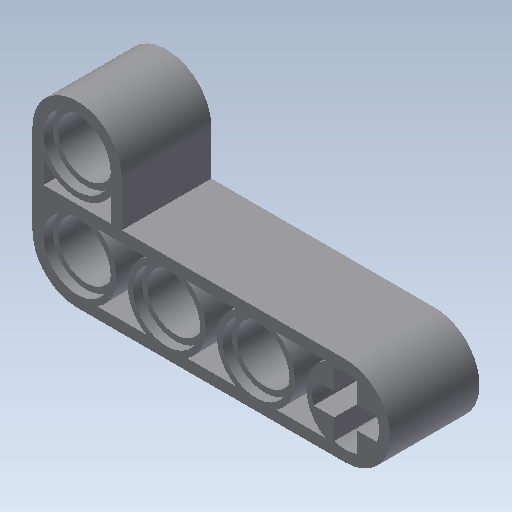
# Autodesk Inventor part: 5MRA Beam
Saved by Autodesk Inventor 2020 (Build 240168000, 168)
## iProperties
Created: 2014-02-14
Part Number: 5MRA Beam
Document SubType Name: Modeling
Designer: Jacob
Density: 1 g/cm^3
Material: Generic
Appearance: Default
Author: Jacob
Autodesk Inventor part; units mm, degrees
ref_plane "YZ Plane" through (0, 0, 0) normal (1, 0, 0) x (0, 1, 0)
ref_plane "XZ Plane" through (0, 0, 0) normal (0, 1, 0) x (-1, 0, 0)
ref_plane "XY Plane" through (0, 0, 0) normal (0, 0, 1) x (1, 0, 0)
sketch "Sketch1" plane through (0, 0, 0) normal (0, 0, 1) x (1, 0, 0)
  arc A0 (-16, 0) -> (-12, -4) centre (-12, 0) ccw
  arc A1 (-8, 8) -> (-16, 8) centre (-12, 8) ccw
  line L0 (-16, 0) -> (-16, 8)
  line L1 (-8, 8) -> (-8, 4)
  arc A2 (12, -4) -> (12, 4) centre (12, 0) ccw
  line L2 (-12, -4) -> (12, -4)
  line L3 (12, 4) -> (-8, 4)
  line L4 (-23.3941, 0) -> (22.5657, 0) projected
  line L5 (0, -8.1941) -> (0, 15.3657) projected
  point P0 (0, 0)
  dimension "d3" = 4
  dimension "d4" = 4
  dimension "d5" = 4
  dimension "d6" = 24
  dimension "d7" = 8
  dimension "d10" = 0
  dimension "d12" = 90
  dimension "d14" = 4
  dimension "d15" = 4
  dimension "d16" = 12
  dimension "d123" = 12
  constraints: 8 end point, 6 point on circle, 3 centre point, 3 tangent, 2 parallel
  measures "d3" radius of A2
  measures "d4" radius of A1
  measures "d5" radius of A0
  measures "d6" distance of A2.centre A0.centre
  measures "d7" distance of A1.centre A0.centre
  measures "d10" distance from line of L4 A0.centre
  measures "d12" angle of L3 L1
  measures "d14" distance between parallel lines of L2 L4
  measures "d15" distance between parallel lines of L4 L3
  measures "d16" distance from line of L5 A1.centre
  measures "d123" distance from line of A2.centre L5
extrude "Extrusion1" add sketch "Sketch1" along normal blind 8
sketch "Sketch13" plane through (0, 0, 8) normal (0, 0, 1) x (1, 0, 0)
  arc A0 (12, -4) -> (12, 4) centre (12, 0) ccw projected
  line L0 (-8, 8) -> (-8, 4) projected
  arc A1 (9.1716, 1) -> (9.1716, -1) centre (12, 0) ccw
  arc A2 (11, -2.8284) -> (13, -2.8284) centre (12, 0) ccw
  arc A3 (14.8284, -1) -> (14.8284, 1) centre (12, 0) ccw
  arc A4 (13, 2.8284) -> (11, 2.8284) centre (12, 0) ccw
  line L1 (14.8284, 1) -> (13, 1)
  line L2 (11, 1) -> (9.1716, 1)
  line L3 (11, -2.8284) -> (11, -1)
  line L4 (11, 1) -> (11, 2.8284)
  line L5 (14.8284, -1) -> (13, -1)
  line L6 (11, -1) -> (9.1716, -1)
  line L7 (13, -2.8284) -> (13, -1)
  line L8 (13, 1) -> (13, 2.8284)
  point P0 (0, 0)
  dimension "d125" = 3
  dimension "d126" = 3
  dimension "d127" = 3
  dimension "d128" = 3
  dimension "d129" = 2
  dimension "d130" = 2
  dimension "d131" = 2
  dimension "d132" = 2
  dimension "d133" = 1
  dimension "d134" = 1
  dimension "d135" = 1
  dimension "d136" = 1
  constraints: 16 end point, 10 parallel, 8 point on circle, 4 centre point, 4 perpendicular, 1 coincident
  measures "d125" radius of A1
  measures "d126" radius of A4
  measures "d127" radius of A2
  measures "d128" radius of A3
  measures "d129" distance between parallel lines of L1 L5
  measures "d130" distance between parallel lines of L8 L4
  measures "d131" distance between parallel lines of L7 L3
  measures "d132" distance between parallel lines of L2 L6
  measures "d133" distance from line of A0.centre L7
  measures "d134" distance from line of L6 A0.centre
  measures "d135" distance from line of L4 A0.centre
  measures "d136" distance from line of L5 A0.centre
extrude "Extrusion13" cut sketch "Sketch13" against normal through all
sketch "Sketch14" plane through (0, 0, 8) normal (0, 0, 1) x (1, 0, 0)
  arc A0 (-16, 0) -> (-12, -4) centre (-12, 0) ccw projected
  line L0 (-8, 4) -> (12, 4) projected
  arc A1 (-8, 8) -> (-16, 8) centre (-12, 8) ccw projected
  circle A2 centre (-12, 0) radius 2.5
  circle A3 centre (-12, 8) radius 2.5
  circle A4 centre (-4, 0) radius 2.5
  circle A5 centre (4, 0) radius 2.5
  point P0 (0, 0)
  dimension "d139" = 5
  dimension "d140" = 5
  dimension "d146" = 8
  constraints: 4 centre point, 2 coincident, 1 horizontal, 4 other
  measures "d139" diameter of A3
  measures "d140" diameter of A2
  measures "d146" distance of A2.centre A4.centre
extrude "Extrusion14" cut sketch "Sketch14" against normal through all
sketch "Sketch15" plane through (0, 0, 8) normal (0, 0, 1) x (1, 0, 0)
  circle A0 centre (4, 0) radius 2.5 projected
  circle A1 centre (-4, 0) radius 2.5 projected
  circle A2 centre (-12, 8) radius 2.5 projected
  circle A3 centre (-12, 0) radius 2.5 projected
  arc A4 (-16, 0) -> (-12, -4) centre (-12, 0) ccw projected
  arc A5 (-8, 8) -> (-16, 8) centre (-12, 8) ccw projected
  circle A6 centre (-12, 0) radius 3
  circle A7 centre (-4, 0) radius 3
  circle A8 centre (4, 0) radius 3
  circle A9 centre (-12, 8) radius 3
  point P0 (0, 0)
  dimension "d150" = 6
  dimension "d151" = 6
  dimension "d152" = 6
  dimension "d153" = 6
  constraints: 4 centre point, 4 coincident
  measures "d150" diameter of A9
  measures "d151" diameter of A6
  measures "d152" diameter of A7
  measures "d153" diameter of A8
extrude "Extrusion15" cut sketch "Sketch15" against normal blind 0.8
sketch "Sketch16" plane through (0, 0, 0) normal (0, 0, -1) x (-1, 0, 0)
  circle A0 centre (-4, 0) radius 2.5 projected
  circle A1 centre (4, 0) radius 2.5 projected
  circle A2 centre (12, 8) radius 2.5 projected
  circle A3 centre (12, 0) radius 2.5 projected
  arc A4 (12, -4) -> (16, 0) centre (12, 0) ccw projected
  arc A5 (16, 8) -> (8, 8) centre (12, 8) ccw projected
  circle A6 centre (12, 8) radius 3
  circle A7 centre (12, 0) radius 3
  circle A8 centre (4, 0) radius 3
  circle A9 centre (-4, 0) radius 3
  point P0 (0, 0)
  dimension "d156" = 6
  dimension "d157" = 6
  dimension "d158" = 6
  dimension "d159" = 6
  constraints: 4 centre point, 4 coincident
  measures "d156" diameter of A7
  measures "d157" diameter of A8
  measures "d158" diameter of A9
  measures "d159" diameter of A6
extrude "Extrusion16" cut sketch "Sketch16" against normal blind 0.8
sketch "Sketch17" plane through (0, 0, 8) normal (0, 0, 1) x (1, 0, 0)
  circle A0 centre (-12, 8) radius 3 projected
  circle A1 centre (-4, 0) radius 3 projected
  circle A2 centre (-12, 0) radius 3 projected
  arc A3 (-16, 0) -> (-12, -4) centre (-12, 0) ccw projected
  line L0 (-8, 4) -> (12, 4) projected
  line L1 (-8, 8) -> (-8, 4) projected
  arc A4 (-8, 8) -> (-16, 8) centre (-12, 8) ccw projected
  arc A5 (-10.1972, -3) -> (-10.1972, 3) centre (-12, 0) ccw
  arc A6 (-5.8028, 3) -> (-5.8028, -3) centre (-4, 0) ccw
  arc A7 (-15, 6.1972) -> (-9, 6.1972) centre (-12, 8) ccw
  line L2 (-10.1972, 3) -> (-5.8028, 3)
  line L3 (-10.1972, -3) -> (-5.8028, -3)
  line L4 (-15, 6.1972) -> (-15, 4)
  line L5 (-9, 6.1972) -> (-9, 4)
  line L6 (-15, 4) -> (-9, 4)
  arc A8 (-2.1972, -3) -> (-2.1972, 3) centre (-4, 0) ccw
  arc A9 (2.1972, 3) -> (2.1972, -3) centre (4, 0) ccw
  line L7 (-2.1972, 3) -> (2.1972, 3)
  line L8 (-2.1972, -3) -> (2.1972, -3)
  arc A10 (5.8028, -3) -> (5.8028, 3) centre (4, 0) ccw
  arc A11 (10.1972, 3) -> (10.1972, -3) centre (12, 0) ccw
  line L9 (5.8028, 3) -> (10.1972, 3)
  line L10 (5.8028, -3) -> (10.1972, -3)
  point P0 (0, 0)
  dimension "d162" = 7
  dimension "d163" = 7
  dimension "d164" = 7
  dimension "d165" = 6
  dimension "d166" = 4
  dimension "d172" = 8
  constraints: 18 end point, 14 point on circle, 7 centre point, 5 tangent, 3 coincident, 2 perpendicular, 1 horizontal, 1 parallel, 20 other
  measures "d162" diameter of A7
  measures "d163" diameter of A5
  measures "d164" diameter of A6
  measures "d165" distance of L4.end L5.end
  measures "d166" distance from line of A0.centre L6
  measures "d172" distance of L2.start L7.start
extrude "Extrusion17" cut sketch "Sketch17" against normal through all contours A5 L2 A6 L3 | A7 L5 L6 L4 | A8 L7 A9 L8 | A10 L9 A11 L10
body "Solid1"
